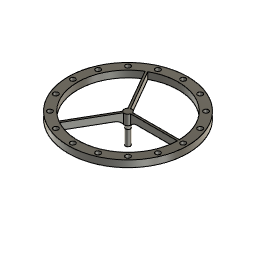
Reaction_Wheel (Autodesk Fusion 360 design; units mm, degrees)
Autodesk Fusion 360 part; units mm, degrees
sketch "스케치1" plane through (0, 0, 0) normal (0, 0, 1) x (1, 0, 0)
  circle A0 centre (0, 0) radius 1.6
  circle A1 centre (0, 0) radius 3.3
  dimension "d1" = 3.2
  dimension "d2" = 6.6
  constraint coincident A0.centre A1.centre
  measures "d1" diameter of A0
  measures "d2" diameter of A1
extrude "돌출1" add sketch "스케치1" along normal blind 30
sketch "스케치2" plane through (0, 0, 30) normal (0, 0, 1) x (-1, 0, 0)
  circle A0 centre (0, 0) radius 80
  circle A1 centre (0, 0) radius 67.5
  circle A2 centre (0, 0) radius 3.3
  line L0 (-3.0247, -1.314) -> (-67.4872, -1.314)
  line L1 (-3.0284, 1.3054) -> (-67.4874, 1.3054)
  circle A3 centre (0, 0) radius 5
  line L2 (2.6503, -1.9624) -> (34.8816, -57.7886)
  line L3 (0.3837, -3.2754) -> (32.6132, -59.0985)
  line L4 (0.3743, 3.2764) -> (32.6056, 59.1027)
  line L5 (2.6447, 1.97) -> (34.8742, 57.7931)
  dimension "d5" = 160
  dimension "d11" = 135
  dimension "d21" = 10
  dimension "d32" = 360
  constraint coincident A0.centre A1.centre
  constraint concentric A1 A3
  constraint coincident A1 L1.end
  constraint horizontal L1
  constraint coincident A1 L0.end
  constraint horizontal L0
  measures "d5" diameter of A0
  measures "d11" diameter of A1
  measures "d21" diameter of A3
extrude "돌출3" add sketch "스케치2" along normal blind 9 contours A0 | A1 A3 L4 L5 | A1 A3 L2 L3 | A2 A3 L4 L5 | A2 A3 L2 L5 | A2 A3 L2 L3 | A1 L0 L1 A3 | A2 L1 A3 L4 | A2 | A2 L0 A3 L3 | A2 L0 L1 A3
sketch "스케치3" plane through (0, 0, 39) normal (0, 0, 1) x (-1, 0, 0)
  circle A0 centre (-74, 0) radius 3.3
  circle A1 centre (-68.3671, -28.3186) radius 3.3
  circle A2 centre (-52.3259, -52.3259) radius 3.3
  circle A3 centre (-28.3186, -68.3671) radius 3.3
  circle A4 centre (0, -74) radius 3.3
  circle A5 centre (28.3186, -68.3671) radius 3.3
  circle A6 centre (52.3259, -52.3259) radius 3.3
  circle A7 centre (68.3671, -28.3186) radius 3.3
  circle A8 centre (74, 0) radius 3.3
  circle A9 centre (68.3671, 28.3186) radius 3.3
  circle A10 centre (52.3259, 52.3259) radius 3.3
  circle A11 centre (28.3186, 68.3671) radius 3.3
  circle A12 centre (0, 74) radius 3.3
  circle A13 centre (-28.3186, 68.3671) radius 3.3
  circle A14 centre (-52.3259, 52.3259) radius 3.3
  circle A15 centre (-68.3671, 28.3186) radius 3.3
  dimension "d33" = 6.6
  dimension "d35" = 360
  measures "d33" diameter of A0
extrude "돌출7" cut sketch "스케치3" against normal through all
fillet "모깎기2" radius 10 1 edges at (-3.0767, -1.1933, 30)
